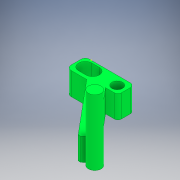
# Autodesk Inventor part: finger_2
Saved by Autodesk Inventor 2018 (Build 220112000, 112)
## iProperties
Created: 2019-01-07
Part Number: finger_2
Material: 一般
Document SubType Name: Modeling
Designer: lowyu
Density: 1 g/cm^3
Appearance: 既定
Author: lowyu
## iProperties of the stored document finger_3D プリント.ipt
Created: 2019-01-08
Part Number: finger_3D プリント
Material: 一般
Document SubType Name: Modeling
Designer: lowyu
Density: 1 g/cm^3
Appearance: 既定
Author: lowyu
Autodesk Inventor part; units mm, degrees
ref_plane "YZ Plane" through (0, 0, 0) normal (1, 0, 0) x (0, 1, 0)
ref_plane "XZ Plane" through (0, 0, 0) normal (0, 1, 0) x (-1, 0, 0)
ref_plane "XY Plane" through (0, 0, 0) normal (0, 0, 1) x (1, 0, 0)
sketch "スケッチ1" plane through (0, 0, 0) normal (0, 0, 1) x (1, 0, 0)
  line L0 (18.3733, -7.7435) -> (14.2723, -7.7348)
  arc A0 (18.3733, -7.7435) -> (20.0717, -6.1303) centre (18.4564, -6.1303) ccw
  line L1 (20.0717, -2.0205) -> (20.0717, -6.1303)
  line L2 (18.408, 0) -> (-1.0303, 0)
  arc A1 (-1.0303, 0) -> (-2.9281, -1.8978) centre (-1.0303, -1.8978) ccw
  line L3 (-2.9281, -1.8978) -> (-2.9281, -6.5862)
  arc A2 (-2.9281, -6.5862) -> (-0.7099, -8.8044) centre (-0.7099, -6.5862) ccw
  arc A3 (26.8795, -33.0792) -> (27.974, -33.1771) centre (27.7186, -29.8656) ccw
  line L4 (29.6865, -31.7299) -> (27.974, -33.1771)
  arc A4 (29.6865, -31.7299) -> (31.4665, -28.292) centre (32.5726, -31.0444) ccw
  line L5 (31.4665, -28.292) -> (14.2723, -7.7348)
  circle A5 centre (16.0858, -4.066) radius 2.5
  line L6 (4.5858, -0.941) -> (1.1333, -0.941)
  arc A6 (4.3798, -7.1842) -> (4.5858, -0.941) centre (4.5858, -4.066) ccw
  line L7 (4.3798, -7.1842) -> (1.0695, -7.1903)
  arc A7 (1.1333, -0.941) -> (1.0695, -7.1903) centre (1.1379, -4.066) ccw
  line L8 (26.8795, -33.0792) -> (6.576, -8.8044)
  line L9 (-0.7099, -8.8044) -> (6.576, -8.8044)
  arc A8 (20.0717, -2.0205) -> (18.408, 0) centre (18.013, -2.0205) ccw
  point P0 (0, 0)
  dimension "d0" = 5
  dimension "d1" = 3.125
  dimension "d17" = 4.8539
  dimension "d24" = 11.5
  dimension "d29" = 14.9479
  dimension "d44" = 4.066
  dimension "d45" = 4.066
  dimension "d46" = 90
  dimension "d47" = 90
  dimension "d48" = 3.125
  dimension "d49" = 3.4479
  constraints: 20 end point, 16 point on circle, 9 centre point, 4 tangent, 2 parallel, 1 coincident, 1 horizontal
  measures "d0" diameter of A5
  measures "d1" radius of A6
  measures "d17" horizontal distance of A4.centre A3.centre
  measures "d24" distance of point (16.086, -4.066) A6.centre
  measures "d29" distance of A7.centre point (16.086, -4.066)
  measures "d44" distance from line of L2 A7.centre
  measures "d45" distance from line of L3 A7.centre
  measures "d48" radius of A7
  measures "d49" distance of A6.centre A7.centre
extrude "押し出し1" add sketch "スケッチ1" along normal blind 10.6
sketch "スケッチ2" plane through (0, 0, 10.6) normal (0, 0, 1) x (1, 0, 0)
  point P0 (0, 0)
sketch "スケッチ3" plane through (0, 0, 10.6) normal (0, 0, 1) x (1, 0, 0)
  arc A0 (29.6865, -31.7299) -> (31.4665, -28.292) centre (32.5726, -31.0444) ccw projected
  arc A1 (31.4665, -28.292) -> (29.6865, -31.7299) centre (32.5726, -31.0444) ccw
  point P0 (0, 0)
  constraints: 2 point on circle, 1 centre point, 1 coincident
extrude "押し出し2" add sketch "スケッチ3" along normal blind 20
equation "\"d45\" = d44"
equation "\"d48\" = d1"
